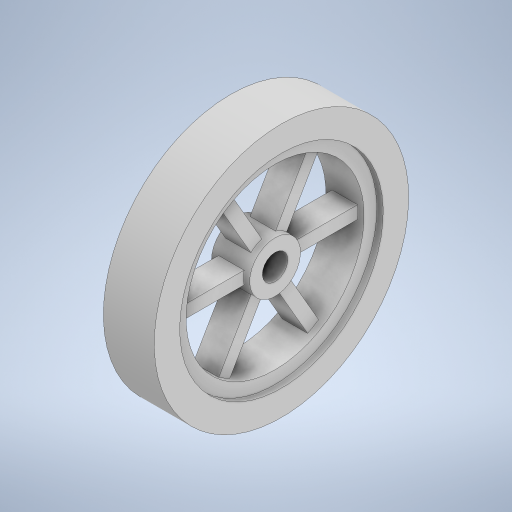
# Autodesk Inventor part: Flywheel
Saved by Autodesk Inventor 2023 (Build 270158000, 158)
## iProperties
Created: 2022-12-28
Part Number: Flywheel
Material: Generic
Document SubType Name: Modeling
Designer: tgr41
Density: 1 g/cm^3
Appearance: Default
Author: tgr41
Autodesk Inventor part; units mm, degrees
ref_plane "YZ Plane" through (0, 0, 0) normal (1, 0, 0) x (0, 1, 0)
ref_plane "XZ Plane" through (0, 0, 0) normal (0, 1, 0) x (-1, 0, 0)
ref_plane "XY Plane" through (0, 0, 0) normal (0, 0, 1) x (1, 0, 0)
sketch "Sketch1" plane through (0, 0, 0) normal (1, 0, 0) x (0, 1, 0)
  circle A0 centre (0, 0) radius 31.75
  circle A1 centre (0, 0) radius 6.35
  line L0 (-1.5875, -6.1484) -> (-1.5875, -22.1682)
  line L1 (1.5875, -6.1484) -> (1.5875, -22.1682)
  circle A2 centre (0, 0) radius 3.175
  circle A3 centre (0, 0) radius 25.4
  circle A4 centre (0, 0) radius 22.225
  line L2 (4.5309, -4.449) -> (18.4045, -12.4589)
  line L3 (6.1184, -1.6994) -> (19.992, -9.7093)
  line L4 (6.1184, 1.6994) -> (19.992, 9.7093)
  line L5 (4.5309, 4.449) -> (18.4045, 12.4589)
  line L6 (1.5875, 6.1484) -> (1.5875, 22.1682)
  line L7 (-1.5875, 6.1484) -> (-1.5875, 22.1682)
  line L8 (-4.5309, 4.449) -> (-18.4045, 12.4589)
  line L9 (-6.1184, 1.6994) -> (-19.992, 9.7093)
  line L10 (-6.1184, -1.6994) -> (-19.992, -9.7093)
  line L11 (-4.5309, -4.449) -> (-18.4045, -12.4589)
  point P0 (-1.5875, 22.1682)
  point P1 (-1.5875, 6.1484)
  point P2 (19.992, -9.7093)
  dimension "d8" = 6.35
  dimension "d11" = 50.8
  dimension "d18" = 63.5
  dimension "d19" = 44.45
  dimension "d22" = 360
  dimension "d28" = 3.175
  constraints: 24 end point, 5 centre point, 5 point on circle, 3 coincident, 1 vertical, 37 other
  measures "d8" diameter of A2
  measures "d11" diameter of A3
  measures "d18" diameter of A0
  measures "d19" diameter of A4
  measures "d28" distance between parallel lines of L1 L0
extrude "Extrusion2" add sketch "Sketch1" along normal mid plane 12.7 contours A0
extrude "Extrusion5" add sketch "Sketch1" along normal mid plane 9.525 contours A1 | A3
extrude "Extrusion6" add sketch "Sketch1" along normal mid plane 6.35 contours A1 L5 A4 L4 | L3 A4 L2 A1 | A1 L7 A4 L6 | L1 A4 L0 A1 | A1 L9 A4 L8 | L11 A4 L10 A1
body "Solid2"
